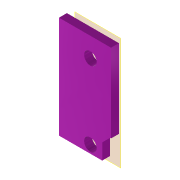
# Autodesk Inventor part: 30_Linear_Stage_NEMA11_baseholder_bayonetmount_objective_autofocus_kes400_camerabracket_underAnAngle_counterplate
Saved by Autodesk Inventor 2022 (Build 260153000, 153)
## iProperties
Created: 2023-06-23
Part Number: 30_Linear_Stage_NEMA11_baseholder_bayonetmount_objective_autofocus_kes400_camerabracket_underAnAngle_counterplate
Material: Generisch
Document SubType Name: Modeling
Designer: diederichbenedict
Density: 1 g/cm^3
Appearance: Glatt - Violett
Author: diederichbenedict
Autodesk Inventor part; units mm, degrees
ref_plane "YZ Plane" through (0, 0, 0) normal (1, 0, 0) x (0, 1, 0)
ref_plane "XZ Plane" through (0, 0, 0) normal (0, 1, 0) x (-1, 0, 0)
ref_plane "XY Plane" through (0, 0, 0) normal (0, 0, 1) x (1, 0, 0)
ref_plane "Arbeitsebene1" through (0, 0, 0) normal (0, 0, 1) x (1, 0, 0)
sketch "Skizze1" plane through (0, 0, 0) normal (0, 0, 1) x (1, 0, 0)
  line L0 (-5.4759, 1.23) -> (2.5633, 4.8092) projected
  line L1 (2.5633, 4.8092) -> (5.3333, -1.4124) projected
  line L2 (5.3333, -1.4124) -> (5.3333, 13) projected
  circle A0 centre (0.0833, 8) radius 1.65
  circle A1 centre (0.0833, -11) radius 1.65
  line L3 (-5.3333, 13) -> (5.3333, 13)
  line L4 (5.3333, 13) -> (5.3333, -13)
  line L5 (5.3333, -13) -> (-5.3333, -13)
  line L6 (-5.3333, -13) -> (-5.3333, 13)
  line L7 (5.3333, -3.5903) -> (-1.8966, -6.8092) projected
  line L8 (-1.8966, -6.8092) -> (-5.4759, 1.23) projected
  line L9 (5.3333, 13) -> (-7.8963, 13) projected
  line L10 (-7.8963, 13) -> (-7.8963, -13) projected
  line L11 (5.3333, -7) -> (5.3333, -3.5903) projected
  line L12 (-7.8963, -13) -> (3.0833, -13) projected
  line L13 (3.0833, -13) -> (3.0833, -9) projected
  line L14 (5.0833, -7) -> (3.0833, -9) projected
  line L15 (5.0833, -7) -> (5.3333, -7) projected
  circle A2 centre (0.0833, -11) radius 1.6 projected
  circle A3 centre (0.0833, 8) radius 1.6 projected
  point P0 (0, 0)
  point P1 (5.3333, -1.4124)
  point P2 (-5.3333, 1.2934)
  point P3 (-2.9167, -13)
  point P4 (-5.3333, 0.9097)
  dimension "d0" = 3.3
  dimension "d1" = 3.3
  constraints: 8 end point, 2 centre point, 2 parallel, 1 horizontal, 1 perpendicular
  measures "d0" diameter of A0
  measures "d1" diameter of A1
extrude "Extrusion1" add sketch "Skizze1" along normal blind 2 contours L8 L6 L12 L10 L9 L0 | L0 L6 L8 | L6 L3 L2 L1 L0 | L0 L1 L4 L7 L8 L6 | L8 L7 L4 L15 L14 L13 L5 L6 | L13 L14 L15 L4 L5 | A0 | A1 | A2 | A3
sketch "Skizze2" plane through (0, 0, 2) normal (0, 0, 1) x (1, 0, 0)
  line L0 (3.0833, -13) -> (3.0833, -9) projected
  line L1 (-2.9167, -13) -> (3.0833, -13) projected
  line L2 (-2.9167, -15) -> (-2.9167, -13) projected
  line L3 (5.0833, -7) -> (5.3333, -7) projected
  line L4 (5.3333, -7) -> (5.3333, 13) projected
  line L5 (3.0833, -9) -> (5.0833, -7) projected
  circle A0 centre (0.0833, 8) radius 1.6 projected
  circle A1 centre (0.3333, -1) radius 4.1 projected
  circle A2 centre (0.0833, -11) radius 1.6 projected
  line L6 (5.3333, -13) -> (5.3333, 13) projected
  line L7 (-7.8963, -13) -> (5.3333, -13) projected
  line L8 (-7.8963, -15) -> (-2.9167, -15) projected
  line L9 (-7.8963, 13) -> (-7.8963, -15) projected
  line L10 (5.3333, 13) -> (-7.8963, 13) projected
  line L11 (5.3333, 13) -> (-7.8963, 13) projected
  line L12 (-7.8963, 13) -> (-7.8963, -13) projected
  point P0 (0, 0)
  point P1 (-5.3333, 13)
  point P2 (-5.3333, 13)
extrude "Extrusion2" cut sketch "Skizze2" against normal blind 10 contours L0 L5 L3 L6 L7 | A0 | A2
